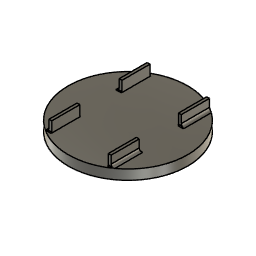
Neck piece bigger attachment v3 v31 (Autodesk Fusion 360 design; units mm, degrees)
Autodesk Fusion 360 part; units mm, degrees
note: some values were not read from the file. Set by a fixed rule: which face or edge a step refers to.
sketch "Sketch1" plane through (0, 0, 0) normal (0, 0, 1) x (1, 0, 0)
  circle A0 centre (0, 0) radius 15.08
  circle A1 centre (0, 0) radius 10.3
  circle A2 centre (0, 0) radius 3.05
  circle A3 centre (0, 0) radius 3.9
  circle A4 centre (0, 0) radius 25
  dimension "d1" = 30.16
  dimension "d2" = 20.6
  dimension "d7" = 6.1
  dimension "d8" = 7.8
  dimension "d9" = 50
  constraint coincident A0.centre A1.centre
  constraint concentric A0 A1
  constraint concentric A0 A2
  constraint concentric A0 A3
  measures "d1" diameter of A0
  measures "d2" diameter of A1
  measures "d7" diameter of A2
  measures "d8" diameter of A3
  measures "d9" diameter of A4
extrude "Extrude1" add sketch "Sketch1" against normal blind 10 contours A0
extrude "Extrude2" add sketch "Sketch1" against normal blind 2 contours A1 | A2 | A3
extrude "Extrude3" add sketch "Sketch1" against normal blind 8 contours A3
extrude "Extrude4" cut 1 faces at (3.5908, -0.3453, -8) along direction (0, 0, 1) blind 7
extrude "Extrude5" add sketch "Sketch1" along normal blind 7 contours A0 | A1 | A2 | A3 | A4
chamfer "Chamfer1" distance 2 angle 45 1 edges at (-9.603, -3.7246, -10)
sketch "Sketch2" plane through (0, 0, 7) normal (0, 0, 1) x (-1, 0, 0)
  circle A0 centre (0, 0) radius 25
  line L0 (20.15, 10) -> (-20.15, 10)
  line L1 (-20.15, 10) -> (-20.15, -10)
  line L2 (-20.15, -10) -> (20.15, -10)
  line L3 (20.15, -10) -> (20.15, 10)
  line L4 (20.15, 10) -> (-20.15, -10) construction
  line L5 (-20.15, 10) -> (20.15, -10) construction
  line L6 (-20.15, 10) -> (-22.15, 10)
  line L7 (-22.15, 10) -> (-22.15, -10)
  line L8 (-22.15, -10) -> (-20.15, -10)
  line L9 (-20.15, -10) -> (-20.15, 10)
  line L10 (20.15, 10) -> (22.15, 10)
  line L11 (22.15, 10) -> (22.15, -10)
  line L12 (22.15, -10) -> (20.15, -10)
  line L13 (20.15, -10) -> (20.15, 10)
  dimension "d17" = 40.3
  dimension "d18" = 20
  dimension "d19" = 2
  dimension "d20" = 20
  dimension "d21" = 2
  dimension "d22" = 20
  constraint horizontal L0
  constraint perpendicular L0 L1
  constraint parallel L0 L2
  constraint parallel L1 L3
  constraint coincident L4 A0.centre
  constraint coincident L5 A0.centre
  constraint coincident A0.centre origin
  constraint horizontal L6
  constraint vertical L7
  constraint horizontal L8
  constraint vertical L9
  constraint horizontal L10
  constraint vertical L11
  constraint horizontal L12
  constraint vertical L13
  measures "d17" distance of L1.end L2.end
  measures "d18" distance of L0.end L1.end
  measures "d19" distance of L0.end L6.end
  measures "d20" distance of L0.end L1.end
  measures "d21" distance of L0.start L10.end
  measures "d22" distance of L0.start L2.end
extrude "Extrude6" add sketch "Sketch2" along normal blind 8 contours L3 L10 L11 L12 L13 | L1 L6 L7 L8 L9
fillet "Fillet1" radius 3 2 edges at (-22.15, 0, 7) (22.15, 0, 7)
fillet "Fillet2" radius 0.5 4 edges at (-21.5314, 10, 7) (21.5314, 10, 7) (-21.5314, -10, 7) (21.5314, -10, 7)
extrude "Extrude7" cut 2 faces at (8.1283, -0.5117, -2) (-0.679, -0.4952, -2) along direction (0, 0, 1) blind 1
extrude "Extrude8" cut 3 faces at (8.1283, -0.5117, -1) (3.5908, -0.3453, -1) (-0.679, -0.4952, -1) along direction (0, 0, 1) blind 0.5
sketch "Sketch3" plane through (0, 0, 7) normal (0, 0, 1) x (-1, 0, 0)
  line L0 (-22.6881, 10.5) -> (-20.15, 10.5)
  line L1 (-20.15, 10.5) -> (-20.15, -10.5)
  line L2 (-20.15, -10.5) -> (-22.6881, -10.5)
  arc A0 (-22.6881, -10.5) -> (22.6881, -10.5) centre (0, 0) ccw
  line L3 (22.6881, -10.5) -> (20.15, -10.5)
  line L4 (20.15, -10.5) -> (20.15, 10.5)
  line L5 (20.15, 10.5) -> (22.6881, 10.5)
  arc A1 (22.6881, 10.5) -> (-22.6881, 10.5) centre (0, 0) ccw
  circle A2 centre (0, 0) radius 42.5
  dimension "d33" = 85
  constraint concentric A0 A2
  measures "d33" diameter of A2
extrude "Extrude9" cut sketch "Sketch3" along normal blind 11
extrude "Extrude10" add sketch "Sketch3" against normal blind 7
sketch "Sketch4" plane through (0, 0, 0) normal (0, 0, 1) x (1, 0, 0)
  circle A0 centre (0, 0) radius 2.975
  circle A1 centre (0, 0) radius 10.6473
  circle A2 centre (0, 0) radius 12.7279
  circle A3 centre (0, 0) radius 3.5
  dimension "d38" = 5.95
  dimension "d49" = 7
  constraint coincident A0.centre A1.centre
  constraint concentric A1 A2
  constraint concentric A2 A3
  measures "d38" diameter of A0
  measures "d49" diameter of A3
extrude "Extrude11" add sketch "Sketch4" against normal blind 6 contours A1 | A2 | A3
fillet "Fillet3" radius 0.5 1 edges at (-2.7737, -1.0758, -6)
fillet "Fillet4" radius 1.5 1 edges at (-14.0595, 5.4532, -10)
extrude "Extrude12" add 1 faces at (7.9737, -0.6844, -6) along direction (0, 0, -1) blind 4
fillet "Fillet5" radius 3 1 edges at (-9.603, -3.7246, -8)
extrude "Extrude13" add sketch "Sketch4" against normal blind 10 contours A3
extrude "Extrude14" cut 1 faces at (7.8089, -0.6595, -10) along direction (0, 0, 1) blind 2
extrude "Extrude15" add 1 faces at (7.8089, -0.6595, -8) along direction (0, 0, -1) blind 2
sketch "Sketch5" plane through (0, 0, 7) normal (0, 0, 1) x (-1, 0, 0)
  circle A0 centre (0, 0) radius 42.5
  line L0 (20.15, -15) -> (-20.15, -15)
  line L1 (-20.15, -15) -> (-20.15, 5)
  line L2 (-20.15, 5) -> (20.15, 5)
  line L3 (20.15, 5) -> (20.15, -15)
  line L4 (20.15, -15) -> (-20.15, 5) construction
  line L5 (-20.15, -15) -> (20.15, 5) construction
  line L6 (-20, -35) -> (-22, -35)
  line L7 (-22, -35) -> (-22, -15)
  line L8 (-22, -15) -> (-20, -15)
  line L9 (-20, -15) -> (-20, -35)
  line L10 (18.3, -35) -> (18.3, -15)
  line L11 (20.3, -15) -> (20.3, -35)
  line L12 (18.3, -15) -> (20.3, -15)
  line L13 (20.3, -35) -> (18.3, -35)
  line L14 (-22, 15) -> (-22, 35)
  line L15 (-20, 35) -> (-20, 15)
  line L16 (-22, 35) -> (-20, 35)
  line L17 (-20, 15) -> (-22, 15)
  line L18 (18.3, 15) -> (18.3, 35)
  line L19 (20.3, 35) -> (20.3, 15)
  line L20 (18.3, 35) -> (20.3, 35)
  line L21 (20.3, 15) -> (18.3, 15)
  point P0 (0, -5)
  dimension "d56" = 40.3
  dimension "d57" = 2
  dimension "d58" = 20
  dimension "d61" = 40.3
  dimension "d62" = 50
  constraint horizontal L0
  constraint perpendicular L0 L1
  constraint parallel L0 L2
  constraint parallel L1 L3
  constraint coincident L4 P0
  constraint coincident L5 P0
  constraint horizontal L6
  constraint vertical L7
  constraint horizontal L8
  constraint vertical L9
  measures "d56" distance of L1.end L2.end
  measures "d57" distance of L6.start L6.end
  measures "d58" distance of L6.start L8.end
extrude "Extrude16" add sketch "Sketch5" along normal blind 7.5 contours L0 L10 L11 L12 L13 | L0 L6 L7 L8 L9 | L14 L15 L16 L17 | L18 L19 L20 L21
extrude "Extrude17" add 2 faces at (22, 28.3333, 9.5) (22, -21.6667, 9.5) along direction (1, 0, 0) blind 1
extrude "Extrude18" add 2 faces at (-20.3, 21.6667, 9.5) (-20.3, -28.3333, 9.5) along direction (-1, 0, 0) blind 1
extrude "Extrude19" cut 2 faces at (20, -28.3333, 9.5) (20, 21.6667, 9.5) along direction (1, 0, 0) blind 1
extrude "Extrude20" cut 2 faces at (-18.3, -21.6667, 9.5) (-18.3, 28.3333, 9.5) along direction (-1, 0, 0) blind 1
fillet "Fillet6" radius 2 4 edges at (-21.3, -25, 7) (-21.3, 25, 7) (23, -25, 7) (23, 25, 7)
fillet "Fillet7" radius 0.5 4 edges at (22.5546, 35, 7) (-21.3, 35, 7) (-21.3, -15, 7) (23, -15, 7)
fillet "Fillet8" radius 0.5 4 edges at (-21.3, 15, 7) (23, 15, 7) (22.5546, -35, 7) (-21.3, -35, 7)
named bodies: "Neck Connetion"
